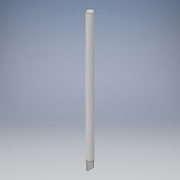
# Autodesk Inventor part: Antenna
Saved by Autodesk Inventor 2018 (Build 220112000, 112)
## iProperties
Created: 2017-12-07
Part Number: Antenna
Material: Generic
Document SubType Name: Modeling
Designer: Andrew
Density: 1 g/cm^3
Appearance: Default
Author: Andrew
Autodesk Inventor part; units mm, degrees
ref_plane "YZ Plane" through (0, 0, 0) normal (1, 0, 0) x (0, 1, 0)
ref_plane "XZ Plane" through (0, 0, 0) normal (0, 1, 0) x (-1, 0, 0)
ref_plane "XY Plane" through (0, 0, 0) normal (0, 0, 1) x (1, 0, 0)
sketch "Sketch1" plane through (0, 0, 0) normal (0, 1, 0) x (-1, 0, 0)
  circle A0 centre (0, 0) radius 3.0353
  line L0 (0.762, 2.9381) -> (-0.762, 2.9381)
  line L1 (-0.762, 2.9381) -> (-0.762, -2.9381)
  line L2 (-0.762, -2.9381) -> (0.762, -2.9381)
  line L3 (0.762, -2.9381) -> (0.762, 2.9381)
  dimension "d0" = 6.0706
  dimension "d1" = 1.524
  constraints: 8 end point, 3 point on circle, 2 parallel, 1 centre point, 1 coincident, 1 horizontal, 1 perpendicular
  measures "d0" diameter of A0
  measures "d1" distance of L1.end L2.end
extrude "Extrusion1" add sketch "Sketch1" along normal blind 127
extrude "Extrusion2" add sketch "Sketch1" against normal blind 7.874 contours L3 L2 L1 L0
body "Solid1"
